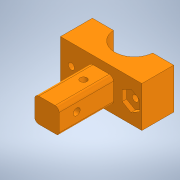
# Autodesk Inventor part: 2_Connettore_inf_sup
Saved by Autodesk Inventor 2020 (Build 240168000, 168)
## iProperties
Created: 2019-10-11
Part Number: 2_Connettore_inf_sup
Material: Generico
Document SubType Name: Modeling
Designer: socci
Density: 1 g/cm^3
Appearance: Arancione
Mass: 37.2193 g
Surface Area: 104.888 cm^2
Volume: 37.2193 cm^3
Author: socci
Autodesk Inventor part; units mm, degrees
ref_plane "YZ Plane" through (0, 0, 0) normal (1, 0, 0) x (0, 1, 0)
ref_plane "XZ Plane" through (0, 0, 0) normal (0, 1, 0) x (-1, 0, 0)
ref_plane "XY Plane" through (0, 0, 0) normal (0, 0, 1) x (1, 0, 0)
sketch "Schizzo1" plane through (0, 0, 0) normal (0, 0, 1) x (1, 0, 0)
  line L0 (7, -9) -> (-6, -9)
  line L1 (-9, -6) -> (-9, 6)
  line L2 (-6, 9) -> (6, 9)
  line L3 (9, 6) -> (9, -7)
  arc A0 (7, -9) -> (9, -7) centre (7, -7) ccw
  arc A1 (-9, -6) -> (-6, -9) centre (-6, -6) ccw
  arc A2 (-6, 9) -> (-9, 6) centre (-6, 6) ccw
  arc A3 (9, 6) -> (6, 9) centre (6, 6) ccw
  point P0 (0, 0)
  point P1 (0, 0)
  point P2 (9, -9)
  point P3 (-9, -9)
  point P4 (-9, 9)
  point P5 (9, 9)
  dimension "d0" = 18
  dimension "d44" = 2
  dimension "d45" = 3
  constraints: 8 end point, 8 point on circle, 8 point on line, 8 tangent, 4 centre point, 2 equal radius, 1 coincident, 9 other
  measures "d0" distance of point (-9, 9) point (9, 9)
  measures "d44" radius of A0
  measures "d45" radius of A1
extrude "Estrusione1" add sketch "Schizzo1" along normal blind 40
sketch "Schizzo2" plane through (0, 0, 0) normal (0, 0, -1) x (-1, 0, 0)
  line L0 (30, -15) -> (-30, -15)
  line L1 (-30, -15) -> (-30, 15)
  line L2 (-30, 15) -> (30, 15)
  line L3 (30, 15) -> (30, -15)
  line L4 (30, -15) -> (-30, 15) construction
  line L5 (-30, -15) -> (30, 15) construction
  point P0 (0, 0)
  dimension "d3" = 60
  dimension "d4" = 30
  constraints: 12 end point, 3 midpoint, 2 parallel, 1 horizontal, 1 perpendicular
  measures "d3" distance of L0.start L0.end
  measures "d4" distance of L0.end L1.end
extrude "Estrusione2" add sketch "Schizzo2" along normal blind 23.5
sketch "Schizzo3" plane through (-30, 15, 0) normal (0, 1, 0) x (1, 0, 0)
  circle A0 centre (30, 24.5) radius 14.5
  line L0 (30, 0) -> (30, 24.5)
  line L1 (60, 23.5) -> (0, 23.5) projected
  line L2 (30, 0) -> (54.5, 0) construction
  dimension "d7" = 29
  dimension "d48" = 24.5
  dimension "d49" = 90
  constraints: 4 end point, 2 perpendicular, 1 centre point, 1 coincident, 1 horizontal
  measures "d7" diameter of A0
  measures "d48" distance of L0.start L0.end
  measures "d49" angle of L2 L0
extrude "Estrusione3" cut sketch "Schizzo3" against normal blind 30
sketch "Schizzo9" plane through (0, 0, 0) normal (0, 0, 1) x (1, 0, 0)
  line L0 (10.5, -10.5) -> (-10.5, -10.5)
  line L1 (-10.5, -10.5) -> (-10.5, 10.5)
  line L2 (-10.5, 10.5) -> (10.5, 10.5)
  line L3 (10.5, 10.5) -> (10.5, -10.5)
  line L4 (13, -13) -> (-13, -13)
  line L5 (-13, -13) -> (-13, 13)
  line L6 (-13, 13) -> (13, 13)
  line L7 (13, 13) -> (13, -13)
  line L8 (-10, 10) -> (-10, -10) projected
  line L9 (10, -10) -> (10, 10) projected
  line L10 (-10, -10) -> (10, -10) projected
  line L11 (9, -9) -> (-9, -9) projected
  point P0 (0, 0)
  point P1 (0, 0)
  point P2 (0, 0)
  dimension "d89" = 21
  dimension "d90" = 26
  constraints: 16 end point, 2 coincident, 18 other
  measures "d89" distance of L2.end L0.start
  measures "d90" distance of L6.end L4.start
extrude "Estrusione4" add sketch "Schizzo9" along normal blind 40
sketch "Schizzo6" plane through (-9, 9, 40) normal (0, 1, 0) x (1, 0, 0)
  line L0 (9, 40) -> (9, 27)
  line L1 (3, 0) -> (16, 0) projected
  line L2 (9, 40) -> (22, 40) construction
  point P0 (0, 0)
  point P1 (18, 0)
  dimension "d27" = 13
  dimension "d28" = 90
  constraints: 4 end point, 2 perpendicular, 1 horizontal
  measures "d27" distance of L0.start L0.end
  measures "d28" angle of L0 L2
hole "Foro2" at (0, 9, 13) direction (0, -1, 0) diameter 5 end through all
sketch "Schizzo7" plane through (-9, -9, 40) normal (-1, 0, 0) x (0, 0, 1)
  line L0 (0, 2) -> (0, 15) projected
  line L1 (0, 9) -> (-13, 9)
  point P0 (-40, 9)
  point P1 (0, 0)
  point P2 (0, 18)
  dimension "d36" = 13
  constraints: 2 end point, 1 horizontal, 1 point on line
  measures "d36" distance of L1.start L1.end
hole "Foro3" at (-9, 0, 27) direction (1, 0, 0) diameter 5 end through all
sketch "Schizzo4" plane through (0, 0, 0) normal (0, 0, 1) x (1, 0, 0)
  line L0 (14.4655, -15) -> (-14.4655, -15) projected
  line L1 (0, -15) -> (0, -8)
  line L2 (0, -8) -> (22, -8)
  line L3 (22, -8) -> (22, 8)
  line L4 (0, -8) -> (-22, -8)
  line L5 (-2.5, -9) -> (-2.5, 9) projected
  line L6 (0, -8) -> (22, -8) construction
  line L7 (-22, -8) -> (-22, 8)
  line L8 (30, -15) -> (-30, -15) projected
  point P0 (0, 0)
  point P1 (0, -15)
  dimension "d73" = 7
  dimension "d74" = 22
  dimension "d75" = 90
  dimension "d76" = 16
  dimension "d77" = 90
  dimension "d78" = 22
  dimension "d79" = 180
  dimension "d80" = 16
  dimension "d81" = 90
  constraints: 12 end point, 4 perpendicular, 2 midpoint, 1 collinear, 1 horizontal, 1 point on line, 1 vertical
  measures "d73" distance of L1.start L1.end
  measures "d74" distance of L1.end L2.end
  measures "d75" angle of L1 L2
  measures "d76" distance of L2.end L3.end
  measures "d77" angle of L3 L2
  measures "d78" distance of L1.end L4.end
  measures "d79" angle of L6 L4
  measures "d80" distance of L4.end L7.end
  measures "d81" angle of L4 L7
hole "Foro4" at (22, -8, 0) at (22, 8, 0) at (-22, -8, 0) at (-22, 8, 0) direction (0, 0, -1) diameter 4.5 end through all clearance for "Vite a testa piana" size "M4" standard "ANSI - Profilo M Metrico"
